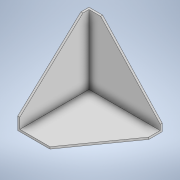
# Autodesk Inventor part: corner_protectipt
Saved by Autodesk Inventor 2022 (Build 260153000, 153)
## iProperties
Created: 2022-08-09
Part Number: corner_protectipt
Material: Generic
Document SubType Name: Modeling
Designer: logic
Density: 1 g/cm^3
Appearance: Default
Author: logic
Autodesk Inventor part; units mm, degrees
ref_plane "YZ Plane" through (0, 0, 0) normal (1, 0, 0) x (0, 1, 0)
ref_plane "XZ Plane" through (0, 0, 0) normal (0, 1, 0) x (-1, 0, 0)
ref_plane "XY Plane" through (0, 0, 0) normal (0, 0, 1) x (1, 0, 0)
sketch "Sketch1" plane through (0, 0, 0) normal (0, 1, 0) x (-1, 0, 0)
  line L0 (17.5, -17.5) -> (-17.5, -17.5) construction
  line L1 (-17.5, -17.5) -> (-17.5, 17.5) construction
  line L2 (-17.5, 17.5) -> (17.5, 17.5) construction
  line L3 (17.5, 17.5) -> (17.5, -17.5) construction
  line L4 (17.5, 17.5) -> (2.6797, 17.5)
  line L5 (2.6797, 17.5) -> (-17.5, -10.9168)
  line L6 (-17.5, -10.9168) -> (-17.5, -17.5)
  line L7 (-17.5, -17.5) -> (17.5, -17.5)
  line L8 (17.5, -17.5) -> (17.5, 17.5)
  point P0 (0, 0)
  dimension "d0" = 35
  dimension "d1" = 35
  dimension "d2" = 17.5
  dimension "d3" = 17.5
  constraints: 18 end point, 2 parallel, 2 point on line, 1 horizontal, 1 perpendicular, 1 vertical
  measures "d0" distance between parallel lines of L1 L3
  measures "d1" distance between parallel lines of L2 L0
  measures "d2" distance from line of point (0, 0) L0
  measures "d3" distance from line of L1 point (0, 0)
extrude "Extrusion1" add sketch "Sketch1" along normal blind 1
sketch "Sketch2" plane through (-17.5, 0, -17.5) normal (-1, 0, 0) x (0, 0, 1)
  line L0 (35, 35) -> (0, 35) construction
  line L1 (0, 35) -> (0, 0) construction
  line L2 (0, 0) -> (35, 0) construction
  line L3 (35, 0) -> (35, 35)
  line L4 (35, 0) -> (35, 6.1852)
  line L5 (35, 6.1852) -> (3.9768, 35)
  line L6 (3.9768, 35) -> (0, 35)
  line L7 (0, 35) -> (0, 0)
  line L8 (0, 0) -> (35, 0)
  point P0 (17.5, 0)
  dimension "d6" = 35
  dimension "d7" = 35
  dimension "d8" = 35
  constraints: 19 end point, 3 horizontal, 2 parallel, 2 perpendicular, 1 coincident
  measures "d6" distance between parallel lines of L3 L1
  measures "d7" distance between parallel lines of L2 L0
  measures "d8" distance between parallel lines of L4 L1
extrude "Extrusion2" add sketch "Sketch2" along normal blind 1
sketch "Sketch3" plane through (17.5, 0, -17.5) normal (0, 0, -1) x (-1, 0, 0)
  line L0 (35, 0) -> (35, 35)
  line L1 (35, 35) -> (29.2734, 35)
  line L2 (29.2734, 35) -> (0, 3.6651)
  line L3 (0, 3.6651) -> (0, 0)
  line L4 (0, 0) -> (35, 0)
  point P0 (17.5, 0)
  dimension "d11" = 35
  dimension "d12" = 35
  constraints: 11 end point, 2 perpendicular, 1 coincident, 1 parallel, 1 vertical
  measures "d11" distance between parallel lines of L4 L1
  measures "d12" distance between parallel lines of L0 L3
extrude "Extrusion3" add sketch "Sketch3" against normal blind 1
body "Solid1"
